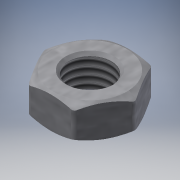
# Autodesk Inventor part: CF-TCA-0001
Saved by Autodesk Inventor 2018.3 (Build 223284000, 284)
## iProperties
Created: 2010-07-22
Part Number: CF-TCA-0001
Document SubType Name: Modeling
Designer: L.Aguerre
Description: TUERCA DIN 934 M3x0.5
Density: 1 g/cm^3
Material: Genérico
Appearance: Metal-acero (inoxidable, cepillado)
BR: -
DES: -
B: -
CCC: -
COC: -
CR: -
GL: -
LGO: -
LT: -
LTO: -
N: -
NG: -
OBR: -
OR: -
PE: -
PL: -
QL: -
QS: -
RPC: -
RU: -
ST: -
STO: -
AI: -
BO: -
BOB: -
CCB: -
CO: -
COB: -
CRB: -
GLO: -
LA: -
LC: -
LG: -
LTC: -
OBR1: -
OOB: -
PC: -
PO: -
POP: -
QLC: -
QLO: -
QR: -
QSC: -
QSO: -
SG: -
SGO: -
STC: -
Linea: -
Maquina: -
Sector: -
ESC.: -
MATERIAL: -
Author: laguerre
Autodesk Inventor part; units mm, degrees
ref_plane "YZ Plane" through (0, 0, 0) normal (1, 0, 0) x (0, 1, 0)
ref_plane "XZ Plane" through (0, 0, 0) normal (0, 1, 0) x (-1, 0, 0)
ref_plane "XY Plane" through (0, 0, 0) normal (0, 0, 1) x (1, 0, 0)
sketch "Sketch17" plane through (0, 0, 0) normal (0, 0, 1) x (1, 0, 0)
  line L0 (-3.0888, 0.15) -> (-1.6743, 2.6)
  line L1 (-1.4145, 2.75) -> (1.4145, 2.75)
  line L2 (1.6743, 2.6) -> (3.0888, 0.15)
  line L3 (3.0888, -0.15) -> (1.6743, -2.6)
  line L4 (1.4145, -2.75) -> (-1.4145, -2.75)
  line L5 (-1.6743, -2.6) -> (-3.0888, -0.15)
  circle A0 centre (0, 0) radius 1.5
  arc A1 (-1.4145, 2.75) -> (-1.6743, 2.6) centre (-1.4145, 2.45) ccw
  arc A2 (1.6743, 2.6) -> (1.4145, 2.75) centre (1.4145, 2.45) ccw
  arc A3 (3.0888, -0.15) -> (3.0888, 0.15) centre (2.829, 0) ccw
  arc A4 (1.4145, -2.75) -> (1.6743, -2.6) centre (1.4145, -2.45) ccw
  arc A5 (-1.6743, -2.6) -> (-1.4145, -2.75) centre (-1.4145, -2.45) ccw
  arc A6 (-3.0888, 0.15) -> (-3.0888, -0.15) centre (-2.829, 0) ccw
  point P0 (-3.1754, 0)
  point P1 (-1.5877, 2.75)
  point P2 (1.5877, 2.75)
  point P3 (3.1754, 0)
  point P4 (1.5877, -2.75)
  point P5 (-1.5877, -2.75)
  dimension "d103" = 5.5
  dimension "d104" = 3
  dimension "d105" = 0.3
  constraints: 12 end point, 12 point on circle, 12 point on line, 12 tangent, 7 centre point, 5 equal radius, 1 coincident, 13 other
  measures "d103" distance between parallel lines of L4 L1
  measures "d104" diameter of A0
  measures "d105" radius of A1
extrude "Extrusion14" add sketch "Sketch17" along normal blind 2.4
sketch "Sketch18" plane through (0, 0, 0) normal (0, 1, 0) x (-1, 0, 0)
  line L0 (-3.0888, 2.4) -> (-1.6743, 2.4) projected
  line L1 (-1.6743, 0) -> (-1.6743, 2.4) projected
  line L2 (-3.0888, 0) -> (-1.6743, 0) projected
  line L3 (-3.0888, 0) -> (-3.0888, 2.4) projected
  line L4 (-1.5, 2.4) -> (1.5, 2.4) projected
  line L5 (1.5, 0) -> (-1.5, 0) projected
  line L6 (1.6743, 2.4) -> (3.0888, 2.4) projected
  line L7 (3.0888, 0) -> (3.0888, 2.4) projected
  line L8 (1.6743, 0) -> (3.0888, 0) projected
  line L9 (1.6743, 0) -> (1.6743, 2.4) projected
  line L10 (0, 2.4) -> (0, 4.8692)
  line L11 (0, 4.8692) -> (0, -2.1161)
  line L12 (1.4145, 0) -> (1.6743, 0) projected
  line L13 (1.4145, 2.4) -> (1.6743, 2.4) projected
  line L14 (1.6743, 0) -> (1.6743, 2.4) projected
  line L15 (1.4145, 0) -> (1.6743, 0) projected
  line L16 (1.4145, 0) -> (1.4145, 2.4) projected
  line L17 (2.5888, 3.8507) -> (2.5888, -1.604) construction
  line L18 (4.0837, 1.5369) -> (4.0837, 3.518)
  line L19 (4.0837, 3.518) -> (2.5888, 3.518)
  line L20 (2.5888, 2.4) -> (2.5888, 3.518)
  line L21 (2.5888, 0) -> (4.2933, 0.9841)
  line L22 (4.2933, 0.9841) -> (4.2933, -0.6301)
  line L23 (4.2933, -0.6301) -> (2.5888, -0.6301)
  line L24 (2.5888, -0.6301) -> (2.5888, 0)
  line L25 (2.5888, 2.4) -> (4.0837, 1.5369)
  dimension "d110" = 30
  dimension "d111" = 30
  dimension "d115" = 0.5
  constraints: 22 end point, 6 point on line, 4 parallel, 3 perpendicular, 2 collinear, 1 midpoint
  measures "d110" angle of L23 L21
  measures "d111" angle of L19 L25
  measures "d115" distance between parallel lines of L7 L17
revolve "Revolution1" cut sketch "Sketch18" angle 360 about axis through (0, 0, 4.8692) along (0, 0, -1) contours L20 L19 L18 L25 L7 L6 | L6 L7 L25 | L21 L7 L8 | L8 L7 L21 L22 L23 L24
thread "Thread3" size "M3x0.5" class "6H" standard "ANSI Metric M Profile" full length
chamfer "Chaflán9" distance 0.2 angle 45 1 edges at (-1.5, 0, 2.4)
chamfer "Chaflán10" distance 0.2 angle 45 1 edges at (-1.5, 0, 0)
